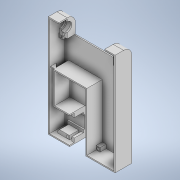
# Autodesk Inventor part: body
Saved by Autodesk Inventor 2022 (Build 260153000, 153)
## iProperties
Created: 2021-01-11
Part Number: body
Material: Generic
Document SubType Name: Modeling
Designer: papa
Density: 1 g/cm^3
Appearance: Default
Author: papa
Autodesk Inventor part; units mm, degrees
ref_plane "YZ Plane" through (0, 0, 0) normal (1, 0, 0) x (0, 1, 0)
ref_plane "XZ Plane" through (0, 0, 0) normal (0, 1, 0) x (-1, 0, 0)
ref_plane "XY Plane" through (0, 0, 0) normal (0, 0, 1) x (1, 0, 0)
sketch "Sketch1" plane through (0, 0, 0) normal (0, 0, 1) x (1, 0, 0)
  line L0 (0, 0) -> (0, 108.5)
  line L1 (0, 108.5) -> (1.5, 108.5)
  line L2 (1.5, 108.5) -> (1.5, 1.5)
  line L3 (1.5, 1.5) -> (27.5, 1.5)
  line L4 (27.5, 1.5) -> (27.5, 0)
  line L5 (27.5, 0) -> (0, 0)
  line L6 (27.5, 36) -> (27.5, 34.5)
  line L7 (27.5, 34.5) -> (6.5, 34.5)
  line L8 (6.5, 34.5) -> (6.5, 76.5)
  line L9 (6.5, 76.5) -> (50, 76.5)
  line L10 (50, 76.5) -> (50, 1.5)
  line L11 (50, 1.5) -> (85, 1.5)
  line L12 (85, 1.5) -> (85, 108.5)
  line L13 (85, 108.5) -> (86.5, 108.5)
  line L14 (86.5, 108.5) -> (86.5, 0)
  line L15 (86.5, 0) -> (48.5, 0)
  line L16 (48.5, 0) -> (48.5, 75)
  line L17 (48.5, 75) -> (8, 75)
  line L18 (8, 75) -> (8, 36)
  line L19 (8, 36) -> (27.5, 36)
  dimension "d0" = 1.5
  dimension "d1" = 1.5
  dimension "d2" = 26
  dimension "d3" = 1.5
  dimension "d4" = 1.5
  dimension "d5" = 1.5
  dimension "d6" = 1.5
  dimension "d7" = 1.5
  dimension "d8" = 1.5
  dimension "d9" = 33
  dimension "d10" = 32
  dimension "d11" = 35
  dimension "d12" = 39
  dimension "d13" = 21
  dimension "d35" = 5
  constraints: 40 end point, 18 perpendicular, 3 collinear, 2 vertical
  measures "d0" distance between parallel lines of L5 L3
  measures "d1" distance between parallel lines of L0 L2
  measures "d2" distance between parallel lines of L2 L4
  measures "d3" distance between parallel lines of L7 L19
  measures "d4" distance between parallel lines of L18 L8
  measures "d5" distance between parallel lines of L9 L17
  measures "d6" distance between parallel lines of L10 L16
  measures "d7" distance between parallel lines of L15 L11
  measures "d8" distance between parallel lines of L14 L12
  measures "d9" distance between parallel lines of L3 L7
  measures "d10" distance between parallel lines of L1 L9
  measures "d11" distance between parallel lines of L12 L10
  measures "d12" distance between parallel lines of L17 L19
  measures "d13" distance between parallel lines of L16 L4
  measures "d35" distance between parallel lines of L2 L8
extrude "Extrusion1" add sketch "Sketch1" along normal blind 20
sketch "Sketch2" plane through (0, 0, 0) normal (0, 0, -1) x (-1, 0, 0)
  line L0 (-48.5, 0) -> (-86.5, 0) projected
  line L1 (0, 108.5) -> (0, 0) projected
  line L2 (-86.5, 0) -> (0, 0)
  line L3 (0, 0) -> (0, 108.5)
  line L4 (0, 108.5) -> (-86.5, 108.5)
  line L5 (-86.5, 108.5) -> (-86.5, 0)
  line L6 (-27.5, 34.5) -> (-27.5, 36) projected
  line L7 (-48.5, 75) -> (-48.5, 0) projected
  line L8 (-27.5, 36) -> (-48.5, 36)
  line L9 (-48.5, 36) -> (-48.5, 0)
  line L10 (-48.5, 0) -> (-27.5, 0)
  line L11 (-27.5, 0) -> (-27.5, 36)
  constraints: 16 end point, 4 parallel, 2 horizontal, 2 perpendicular
extrude "Extrusion2" add sketch "Sketch2" along normal blind 1.5 contours L0 L5 L4 L1 L2 L11 L6 L8 L7
sketch "Sketch3" plane through (6.5, 76.5, 20) normal (0, 1, 0) x (1, 0, 0)
  line L0 (0, 3.5) -> (0, 1.5)
  line L1 (0, 1.5) -> (-5, 1.5)
  line L2 (-5, 1.5) -> (-5, 8.5)
  line L3 (-5, 8.5) -> (0, 3.5)
  line L4 (-5, 20) -> (-5, 0) projected
  line L5 (0, 20) -> (0, 0) projected
  line L6 (21, 0) -> (-5, 0) projected
  dimension "d21" = 1.5
  dimension "d22" = 45
  dimension "d23" = 2
  constraints: 8 end point, 2 collinear, 1 horizontal
  measures "d21" distance between parallel lines of L6 L1
  measures "d22" angle of L2 L3
  measures "d23" distance of L0.start L0.end
extrude "Extrusion3" add sketch "Sketch3" against normal blind 1.5 contours L0 L1 L2 L3
sketch "Sketch4" plane through (0, 0, 0) normal (0, 0, 1) x (1, 0, 0)
  line L0 (6.5, 34.5) -> (27.5, 34.5) projected
  line L1 (6.5, 34.5) -> (27.5, 34.5)
  line L2 (27.5, 34.5) -> (27.5, 26)
  line L3 (27.5, 26) -> (6.5, 26)
  line L4 (6.5, 26) -> (6.5, 34.5)
  line L5 (27.5, 1.5) -> (1.5, 1.5) projected
  line L6 (6.5, 10) -> (27.5, 10)
  line L7 (27.5, 10) -> (27.5, 1.5)
  line L8 (27.5, 1.5) -> (6.5, 1.5)
  line L9 (6.5, 1.5) -> (6.5, 10)
  point P0 (0, 0)
  point P1 (6.5, 1.5)
  dimension "d26" = 16
  constraints: 16 end point, 4 parallel, 2 horizontal, 2 perpendicular, 1 collinear, 1 point on line
  measures "d26" distance between parallel lines of L6 L3
extrude "Extrusion4" add sketch "Sketch4" along normal blind 2
sketch "Sketch5" plane through (0, 0, 2) normal (0, 0, 1) x (1, 0, 0)
  line L0 (6.5, 34.5) -> (6.5, 26) projected
  line L1 (6.5, 34.5) -> (21.5, 34.5)
  line L2 (21.5, 34.5) -> (21.5, 29.5)
  line L3 (21.5, 29.5) -> (6.5, 29.5)
  line L4 (6.5, 29.5) -> (6.5, 34.5)
  line L5 (6.5, 1.5) -> (1.5, 1.5) projected
  line L6 (6.5, 1.5) -> (21.5, 1.5)
  line L7 (21.5, 1.5) -> (21.5, 6.5)
  line L8 (21.5, 6.5) -> (6.5, 6.5)
  line L9 (6.5, 6.5) -> (6.5, 1.5)
  line L10 (27.5, 1.5) -> (1.5, 1.5) projected
  line L11 (27.5, 1.5) -> (24.5, 1.5)
  line L12 (24.5, 1.5) -> (24.5, 6.5)
  line L13 (24.5, 6.5) -> (27.5, 6.5)
  line L14 (27.5, 6.5) -> (27.5, 1.5)
  line L15 (27.5, 34.5) -> (24.5, 34.5)
  line L16 (24.5, 34.5) -> (24.5, 29.5)
  line L17 (24.5, 29.5) -> (27.5, 29.5)
  line L18 (27.5, 29.5) -> (27.5, 34.5)
  line L19 (1.5, 1.5) -> (1.5, 108.5) projected
  point P0 (0, 0)
  point P1 (24.5, 1.5)
  point P2 (6.5, 29.5)
  dimension "d29" = 23
  dimension "d30" = 23
  dimension "d31" = 3
  dimension "d32" = 20
  constraints: 32 end point, 8 parallel, 4 horizontal, 4 perpendicular, 3 collinear, 1 point on line
  measures "d29" distance between parallel lines of L8 L3
  measures "d30" distance between parallel lines of L13 L17
  measures "d31" distance between parallel lines of L16 L2
  measures "d32" distance between parallel lines of L19 L2
extrude "Extrusion5" add sketch "Sketch5" along normal blind 12
sketch "Sketch6" plane through (1.5, 108.5, 0) normal (0, 1, 0) x (1, 0, 0)
  line L0 (85, -20) -> (85, 1.5)
  line L1 (85, 1.5) -> (71.5, 1.5)
  line L2 (71.5, 1.5) -> (71.5, -9)
  line L3 (71.5, -9) -> (73.5, -9)
  line L4 (73.5, -9) -> (73.5, 0)
  line L5 (73.5, 0) -> (83.5, 0)
  line L6 (83.5, 0) -> (83.5, -20)
  line L7 (83.5, -20) -> (85, -20)
  line L8 (85, -20) -> (83.5, -20) projected
  line L9 (-1.5, 1.5) -> (85, 1.5) projected
  line L10 (85, 1.5) -> (85, -20) projected
  line L11 (-1.5, -20) -> (-1.5, 1.5)
  line L12 (-1.5, 1.5) -> (12, 1.5)
  line L13 (12, 1.5) -> (12, -9)
  line L14 (12, -9) -> (10, -9)
  line L15 (10, -9) -> (10, 0)
  line L16 (10, 0) -> (0, 0)
  line L17 (0, 0) -> (0, -20)
  line L18 (0, -20) -> (-1.5, -20)
  line L19 (0, -20) -> (-1.5, -20) projected
  line L20 (-1.5, 1.5) -> (-1.5, -20) projected
  dimension "d36" = 1.5
  dimension "d37" = 1.5
  dimension "d38" = 2
  dimension "d39" = 10
  dimension "d41" = 1.5
  dimension "d42" = 1.5
  dimension "d43" = 2
  dimension "d44" = 10
  dimension "d54" = 10.5
  constraints: 32 end point, 14 perpendicular, 7 collinear, 2 vertical
  measures "d36" distance between parallel lines of L6 L0
  measures "d37" distance between parallel lines of L1 L5
  measures "d38" distance between parallel lines of L2 L4
  measures "d39" distance between parallel lines of L6 L4
  measures "d41" distance between parallel lines of L11 L17
  measures "d42" distance between parallel lines of L12 L16
  measures "d43" distance between parallel lines of L13 L15
  measures "d44" distance between parallel lines of L15 L17
  measures "d54" distance between parallel lines of L3 L9
extrude "Extrusion6" add sketch "Sketch6" along normal blind 22
sketch "Sketch7" plane through (1.5, 130.5, 0) normal (0, 1, 0) x (1, 0, 0)
  line L0 (26, 1.5) -> (-1.5, 1.5) projected
  line L1 (-1.5, -20) -> (-1.5, 1.5) projected
  line L2 (12, 1.5) -> (-1.5, 1.5)
  line L3 (-1.5, 1.5) -> (-1.5, -20)
  line L4 (-1.5, -20) -> (12, -20)
  line L5 (12, -20) -> (12, 1.5)
  line L6 (71.5, 1.5) -> (71.5, -9) projected
  line L7 (47, -20) -> (85, -20) projected
  line L8 (71.5, 1.5) -> (85, 1.5)
  line L9 (85, 1.5) -> (85, -20)
  line L10 (85, -20) -> (71.5, -20)
  line L11 (71.5, -20) -> (71.5, 1.5)
  point P0 (-1.5, 0)
  point P1 (71.5, -9)
  constraints: 16 end point, 4 parallel, 2 horizontal, 2 perpendicular, 1 point on line
extrude "Extrusion7" add sketch "Sketch7" along normal blind 1.5
fillet "Fillet1" radius 9 2 edges at (6.5, 130.5, 0) (80, 130.5, 0)
sketch "Sketch8" plane through (73, 108.5, 0) normal (-1, 0, 0) x (0, 0, 1)
  circle A0 centre (9, 13) radius 3.5
  line L0 (-1.5, 23.5) -> (20, 23.5) projected
  line L1 (-1.5, -108.5) -> (-1.5, 23.5) projected
  point P0 (0, -108.5)
  point P1 (9, 26.5)
  point P2 (-1.5, 16)
  dimension "d51" = 7
  dimension "d53" = 10.5
  dimension "d68" = 10.5
  constraints: 1 centre point, 1 other
  measures "d51" diameter of A0
  measures "d53" distance from line of L1 A0.centre
extrude "Extrusion8" cut sketch "Sketch8" against normal blind 2
sketch "Sketch11" plane through (0, 0, 0) normal (0, 0, 1) x (1, 0, 0)
  line L0 (85, 115.25) -> (82, 115.25)
  line L1 (82, 115.25) -> (82, 120)
  line L2 (82, 120) -> (85, 120)
  line L3 (85, 120) -> (85, 115.25)
  line L4 (85, 127.75) -> (82, 127.75)
  line L5 (82, 127.75) -> (82, 123)
  line L6 (82, 123) -> (85, 123)
  line L7 (85, 123) -> (85, 127.75)
  line L8 (75, 108.5) -> (75, 130.5) projected
  line L9 (75, 115.25) -> (78, 115.25)
  line L10 (78, 115.25) -> (78, 112.5)
  line L11 (78, 112.5) -> (75, 112.5)
  line L12 (75, 112.5) -> (75, 115.25)
  line L13 (75, 127.75) -> (78, 127.75)
  line L14 (78, 127.75) -> (78, 130.5)
  line L15 (78, 130.5) -> (75, 130.5)
  line L16 (75, 130.5) -> (75, 127.75)
  line L17 (75, 118) -> (73, 118) projected
  line L18 (85, 1.5) -> (85, 130.5) projected
  point P0 (0, 0)
  dimension "d59" = 12.5
  dimension "d61" = 7
  dimension "d62" = 3
  dimension "d65" = 3
  dimension "d71" = 2.75
  constraints: 32 end point, 8 parallel, 5 collinear, 5 point on line, 4 horizontal, 4 perpendicular
  measures "d59" distance between parallel lines of L9 L13
  measures "d61" distance between parallel lines of L8 L1
  measures "d62" distance between parallel lines of L12 L10
  measures "d65" distance between parallel lines of L2 L6
  measures "d71" distance between parallel lines of L9 L17
extrude "Extrusion9" add sketch "Sketch11" along normal up to surface (9 mm away)
sketch "Sketch12" plane through (0, 0, 0) normal (0, 0, 1) x (1, 0, 0)
  line L0 (75, 115.25) -> (78, 115.25) projected
  line L1 (82, 123) -> (82, 127.75) projected
  line L2 (75, 115.25) -> (82, 115.25)
  line L3 (82, 115.25) -> (82, 127.75)
  line L4 (82, 127.75) -> (75, 127.75)
  line L5 (75, 127.75) -> (75, 115.25)
  point P0 (0, 0)
  constraints: 8 end point, 2 parallel, 1 horizontal, 1 perpendicular
extrude "Extrusion10" add sketch "Sketch12" along normal blind 2.75
sketch "Sketch13" plane through (0, 0, 0) normal (0, 0, 1) x (1, 0, 0)
  point P0 (0, 0)
sketch "Sketch14" plane through (0, 0, 0) normal (0, 0, 1) x (1, 0, 0)
  line L0 (11.5, 108.5) -> (5.5, 108.5)
  line L1 (5.5, 108.5) -> (5.5, 130.5)
  line L2 (5.5, 130.5) -> (11.5, 130.5)
  line L3 (11.5, 130.5) -> (11.5, 108.5)
  line L4 (1.5, 130.5) -> (13.5, 130.5) projected
  line L5 (11.5, 108.5) -> (11.5, 130.5) projected
  point P0 (0, 0)
  dimension "d72" = 6
  dimension "d73" = 22
  constraints: 8 end point, 2 collinear, 2 parallel, 1 horizontal, 1 perpendicular
  measures "d72" distance of L1.end L2.end
  measures "d73" distance between parallel lines of L2 L0
extrude "Extrusion11" add sketch "Sketch14" along normal up to surface (9 mm away)
sketch "Sketch15" plane through (5.5, 108.5, 0) normal (-1, 0, 0) x (0, 0, 1)
  line L0 (9, 0) -> (9, 22) projected
  circle A0 centre (9, 13) radius 8
  point P0 (0, -108.5)
  point P1 (9, 21)
  point P2 (9, 5)
  dimension "d76" = 16
  constraints: 1 centre point, 1 point on line
  measures "d76" diameter of A0
extrude "Extrusion12" cut sketch "Sketch15" against normal blind 6 contours A0 L0 picked at (6.3528, 13.3214)
sketch "Sketch16" plane through (0, 0, 0) normal (0, 0, 1) x (1, 0, 0)
  line L0 (5.5, 108.5) -> (3.5, 108.5)
  line L1 (3.5, 108.5) -> (3.5, 130.5)
  line L2 (3.5, 130.5) -> (5.5, 130.5)
  line L3 (5.5, 130.5) -> (5.5, 108.5)
  line L4 (13.5, 108.5) -> (5.5, 108.5) projected
  line L5 (13.5, 130.5) -> (5.5, 130.5) projected
  line L6 (5.5, 108.5) -> (5.5, 121.5) projected
  point P0 (0, 0)
  dimension "d126" = 2
  constraints: 8 end point, 3 collinear, 2 parallel, 1 horizontal, 1 perpendicular
  measures "d126" distance between parallel lines of L6 L1
extrude "Extrusion13" add sketch "Sketch16" along normal up to surface (9 mm away)
sketch "Sketch17" plane through (13.5, 108.5, 9) normal (1, 0, 0) x (0, 0, -1)
  arc A0 (0, 9.5) -> (0, 16.5) centre (0, 13) ccw projected
  circle A1 centre (0, 13) radius 6
  point P0 (9, -108.5)
  constraints: 1 centre point, 1 coincident
extrude "Extrusion14" cut sketch "Sketch17" against normal up to surface (10 mm away)
move faces "Move1" translate (3, 0, 0) faces at (75, 111.1667, 6)
sketch "Sketch18" plane through (0, 0, 0) normal (0, 0, 1) x (1, 0, 0)
  line L0 (85, 115.25) -> (85, 1.5) projected
  line L1 (85, 81.5) -> (80, 81.5)
  line L2 (80, 81.5) -> (80, 71.5)
  line L3 (80, 71.5) -> (85, 71.5)
  line L4 (85, 71.5) -> (85, 81.5)
  line L5 (50, 76.5) -> (6.5, 76.5) projected
  line L6 (6.5, 103.5) -> (1.5, 103.5)
  line L7 (1.5, 103.5) -> (1.5, 108.5)
  line L8 (1.5, 108.5) -> (6.5, 108.5)
  line L9 (6.5, 108.5) -> (6.5, 103.5)
  line L10 (1.5, 1.5) -> (1.5, 130.5) projected
  line L11 (13.5, 108.5) -> (3.5, 108.5) projected
  line L12 (50, 1.5) -> (50, 76.5) projected
  line L13 (50, 1.5) -> (55, 1.5)
  line L14 (55, 1.5) -> (55, 6.5)
  line L15 (55, 6.5) -> (50, 6.5)
  line L16 (50, 6.5) -> (50, 1.5)
  point P0 (0, 0)
  point P1 (5.5, 108.5)
  dimension "d86" = 5
  dimension "d87" = 10
  dimension "d88" = 5
  dimension "d89" = 5
  dimension "d90" = 5
  dimension "d91" = 5
  dimension "d92" = 5
  constraints: 24 end point, 6 parallel, 3 horizontal, 3 perpendicular, 2 collinear, 1 point on line
  measures "d86" distance of L3.end L2.end
  measures "d87" distance of L2.end L1.end
  measures "d88" distance between parallel lines of L3 L5
  measures "d89" distance of L7.end L8.end
  measures "d90" distance of L6.end L7.end
  measures "d91" distance of L15.end L14.end
  measures "d92" distance of L14.end L13.end
extrude "Extrusion15" add sketch "Sketch18" along normal blind 8
sketch "Sketch19" plane through (0, 0, 0) normal (0, 0, 1) x (1, 0, 0)
  circle A0 centre (52.5, 4) radius 1.75
  circle A1 centre (19, 4) radius 1.75
  circle A2 centre (9, 32) radius 1.75
  circle A3 centre (82.5, 74) radius 1.75
  circle A4 centre (82.5, 79) radius 1.75
  circle A5 centre (4, 106) radius 1.75
  circle A6 centre (8.5, 111) radius 1.75
  circle A7 centre (75.5, 111) radius 1.75
  line L0 (80, 71.5) -> (85, 71.5) projected
  line L1 (85, 81.5) -> (80, 81.5) projected
  line L2 (85, 1.5) -> (85, 130.5) projected
  line L3 (73, 108.5) -> (73, 118) projected
  line L4 (73, 108.5) -> (78, 108.5) projected
  line L5 (13.5, 108.5) -> (5.5, 108.5) projected
  line L6 (13.5, 108.5) -> (13.5, 130.5) projected
  line L7 (21.5, 1.5) -> (21.5, 6.5) projected
  line L8 (21.5, 6.5) -> (6.5, 6.5) projected
  line L9 (6.5, 34.5) -> (6.5, 29.5) projected
  line L10 (6.5, 34.5) -> (27.5, 34.5) projected
  line L11 (85, 1.5) -> (50, 1.5) projected
  line L12 (50, 1.5) -> (50, 76.5) projected
  line L13 (1.5, 1.5) -> (1.5, 130.5) projected
  point P0 (0, 0)
  point P1 (3.5, 108.5)
  point P2 (13.5, 115.5)
  dimension "d100" = 3.5
  dimension "d101" = 3.5
  dimension "d102" = 3.5
  dimension "d103" = 3.5
  dimension "d104" = 3.5
  dimension "d105" = 3.5
  dimension "d106" = 3.5
  dimension "d107" = 3.5
  dimension "d108" = 2.5
  dimension "d109" = 2.5
  dimension "d110" = 2.5
  dimension "d111" = 2.5
  dimension "d112" = 2.5
  dimension "d113" = 2.5
  dimension "d114" = 2.5
  dimension "d115" = 5
  dimension "d116" = 2.5
  dimension "d117" = 2.5
  dimension "d118" = 2.5
  dimension "d119" = 2.5
  dimension "d120" = 2.5
  dimension "d121" = 2.5
  dimension "d124" = 2.5
  dimension "d125" = 2.5
  constraints: 8 centre point
  measures "d100" diameter of A0
  measures "d101" diameter of A1
  measures "d102" diameter of A2
  measures "d103" diameter of A3
  measures "d104" diameter of A4
  measures "d105" diameter of A5
  measures "d106" diameter of A6
  measures "d107" diameter of A7
  measures "d108" distance from line of L0 A3.centre
  measures "d109" distance from line of L1 A4.centre
  measures "d110" distance from line of L2 A4.centre
  measures "d111" distance from line of L2 A3.centre
  measures "d112" distance from line of L3 A7.centre
  measures "d113" distance from line of L4 A7.centre
  measures "d114" distance from line of L5 A6.centre
  measures "d115" distance from line of L6 A6.centre
  measures "d116" distance from line of L7 A1.centre
  measures "d117" distance from line of L8 A1.centre
  measures "d118" distance from line of L9 A2.centre
  measures "d119" distance from line of L10 A2.centre
  measures "d120" distance from line of L11 A0.centre
  measures "d121" distance from line of L12 A0.centre
  measures "d124" distance from line of L13 A5.centre
  measures "d125" distance from line of L5 A5.centre
extrude "Extrusion16" cut sketch "Sketch19" along normal through all both and the other way through all
fillet "Fillet3" radius 10.5 2 edges at (79.75, 132, -1.5) (6.75, 132, -1.5)
chamfer "Chamfer1" distance 2 angle 45 1 edges at (6.5, 6.5, 8)
body "Solid1"
